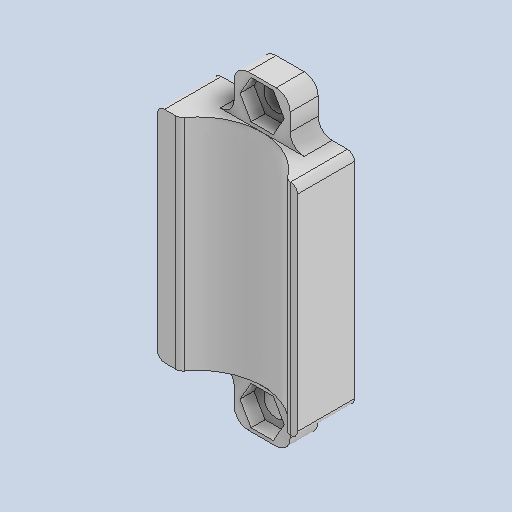
# Autodesk Inventor part: baterry_holder
Saved by Autodesk Inventor 2023 (Build 270158000, 158)
## iProperties
Created: 2023-07-29
Part Number: baterry_holder
Material: Ogólny
Document SubType Name: Modeling
Designer: Kamil
Density: 1 g/cm^3
Appearance: Domyślna
Author: Kamil
Autodesk Inventor part; units mm, degrees
ref_plane "YZ Plane" through (0, 0, 0) normal (1, 0, 0) x (0, 1, 0)
ref_plane "XZ Plane" through (0, 0, 0) normal (0, 1, 0) x (-1, 0, 0)
sketch "Szkic1" plane through (0, 0, 0) normal (0, 0, 1) x (1, 0, 0)
  line L0 (-47.8749, 26.935) -> (-29.4749, 26.935) projected
  line L1 (-47.2702, -7.5558) -> (-30.0796, -7.5558) projected
  line L2 (-29.4749, 23.0223) -> (-29.4749, -7.065)
  line L3 (-47.8749, 23.0223) -> (-47.8749, -7.065)
  line L4 (-47.1734, 27.6365) -> (-30.1764, 27.6365) projected
  line L5 (-47.1749, -7.765) -> (-30.1749, -7.765) projected
  line L6 (-29.4749, 27.6365) -> (-47.8749, 27.6365)
  line L7 (-47.8749, 27.6365) -> (-47.8749, -7.765)
  line L8 (-47.8749, -7.765) -> (-29.4749, -7.765)
  line L9 (-29.4749, -7.765) -> (-29.4749, 27.6365)
  line L10 (-29.4749, 27.6365) -> (-47.8749, 27.6365)
  line L11 (-47.8749, 27.6365) -> (-47.8749, 23.6365)
  line L12 (-47.8749, 23.6365) -> (-29.4749, 23.6365)
  line L13 (-29.4749, 23.6365) -> (-29.4749, 27.6365)
  point P0 (0, 0)
  point P1 (-47.8749, -7.065)
  point P2 (-29.4749, -7.065)
  dimension "d0" = 4
  constraints: 20 end point, 4 parallel, 2 horizontal, 2 perpendicular, 2 vertical, 1 point on line, 4 other
  measures "d0" distance of L11.end L10.end
ref_plane "Płaszczyzna konstrukcyjna1" through (-46.6386, 28.6013, 8.141) normal (0, 0, -1) x (0, 1, 0)
extrude "Wyciągnięcie proste1" add sketch "Szkic1" along normal up to surface (8.141 mm away) contours L12 L9 L2 L8 L5 L7 L3
sketch "Szkic2" plane through (-47.8749, -7.765, 0) normal (0, -1, 0) x (1, 0, 0)
  circle A0 centre (9.2, 13.221) radius 9.2 projected
  line L0 (0, 8.141) -> (18.4, 8.141) projected
  point P0 (47.8749, 0)
  point P1 (16.8703, 8.141)
  point P2 (1.5297, 8.141)
extrude "Wyciągnięcie proste2" cut sketch "Szkic2" against normal through all contours L0 A0 picked at (10.6511, 7.1327)
sketch "Szkic3" plane through (0, 0, 0) normal (0, 0, -1) x (-1, 0, 0)
  line L0 (47.8749, 23.6365) -> (47.8749, -7.765) projected
  line L1 (29.4749, 23.6365) -> (47.8749, 23.6365) projected
  line L2 (29.4749, -7.765) -> (29.4749, 23.6365) projected
  line L3 (47.8749, -7.765) -> (29.4749, -7.765) projected
  line L4 (42.6749, 30.1365) -> (34.6749, 30.1365)
  line L5 (34.6749, 30.1365) -> (34.6749, 23.6365)
  line L6 (34.6749, 23.6365) -> (42.6749, 23.6365)
  line L7 (42.6749, 23.6365) -> (42.6749, 30.1365)
  line L8 (42.6749, -7.765) -> (34.6749, -7.765)
  line L9 (34.6749, -7.765) -> (34.6749, -14.265)
  line L10 (34.6749, -14.265) -> (42.6749, -14.265)
  line L11 (42.6749, -14.265) -> (42.6749, -7.765)
  point P0 (0, 0)
  point P1 (38.6749, 23.6365)
  point P2 (38.6749, 23.6365)
  dimension "d7" = 8
  dimension "d8" = 6.5
  dimension "d9" = 6.5
  constraints: 16 end point, 4 parallel, 2 horizontal, 2 midpoint, 2 perpendicular, 1 coincident, 1 collinear, 1 point on line
  measures "d7" distance of L6.end L5.end
  measures "d8" distance of L5.end L4.end
  measures "d9" distance of L9.end L8.end
extrude "Wyciągnięcie proste3" add sketch "Szkic3" against normal blind 2 contours L1 L5 L4 L7 | L11 L10 L9 L3
sketch "Szkic4" plane through (0, 0, 2) normal (0, 0, 1) x (1, 0, 0)
  line L0 (-34.6749, 23.6365) -> (-34.6749, 30.1365) projected
  line L1 (-34.6749, 30.1365) -> (-42.6749, 30.1365) projected
  line L2 (-42.6749, 30.1365) -> (-42.6749, 23.6365) projected
  line L3 (-34.6749, 23.6365) -> (-42.6749, 23.6365) projected
  line L4 (-42.6749, -7.765) -> (-42.6749, -14.265) projected
  line L5 (-42.6749, -14.265) -> (-34.6749, -14.265) projected
  line L6 (-34.6749, -14.265) -> (-34.6749, -7.765) projected
  line L7 (-42.6749, -7.765) -> (-34.6749, -7.765) projected
  point P0 (0, 0)
  point P1 (-38.6749, 26.8865)
  point P2 (-38.6749, -11.015)
hole "Otwór1" at (-38.6749, 26.8865, 2) at (-38.6749, -11.015, 2) direction (0, 0, -1) diameter 3.5 end through all
sketch "Szkic5" plane through (0, 0, 2) normal (0, 0, 1) x (1, 0, 0)
  circle A0 centre (-38.6749, 26.8865) radius 1.75 projected
  line L0 (-34.6749, 23.6365) -> (-34.6749, 30.1365) projected
  line L1 (-34.6749, 30.1365) -> (-42.6749, 30.1365) projected
  line L2 (-42.6749, 30.1365) -> (-42.6749, 23.6365) projected
  line L3 (-34.6749, 23.6365) -> (-42.6749, 23.6365) projected
  circle A1 centre (-38.6749, -11.015) radius 1.75 projected
  line L4 (-42.6749, -7.765) -> (-42.6749, -14.265) projected
  line L5 (-42.6749, -14.265) -> (-34.6749, -14.265) projected
  line L6 (-34.6749, -14.265) -> (-34.6749, -7.765) projected
  line L7 (-42.6749, -7.765) -> (-34.6749, -7.765) projected
  circle A2 centre (-38.6749, 26.8865) radius 2.75
  circle A3 centre (-38.6749, -11.015) radius 2.75
  line L8 (-37.0872, 29.6365) -> (-35.4995, 26.8865)
  line L9 (-35.4995, 26.8865) -> (-37.0872, 24.1365)
  line L10 (-37.0872, 24.1365) -> (-40.2626, 24.1365)
  line L11 (-40.2626, 24.1365) -> (-41.8503, 26.8865)
  line L12 (-41.8503, 26.8865) -> (-40.2626, 29.6365)
  line L13 (-40.2626, 29.6365) -> (-37.0872, 29.6365)
  line L14 (-40.2626, -13.765) -> (-41.8503, -11.015)
  line L15 (-41.8503, -11.015) -> (-40.2626, -8.265)
  line L16 (-40.2626, -8.265) -> (-37.0872, -8.265)
  line L17 (-37.0872, -8.265) -> (-35.4995, -11.015)
  line L18 (-35.4995, -11.015) -> (-37.0872, -13.765)
  line L19 (-37.0872, -13.765) -> (-40.2626, -13.765)
  point P0 (0, 0)
  point P1 (-38.6749, 29.6365)
  point P2 (-38.6749, -13.765)
  dimension "d19" = 5.5
  dimension "d20" = 5.5
  constraints: 24 end point, 4 coincident, 2 midpoint, 2 vertical alignment, 30 other
extrude "Wyciągnięcie proste4" add sketch "Szkic5" along normal blind 2 contours L3 L2 L1 L0 | L7 L6 L5 L4
sketch "Szkic6" plane through (-47.8749, -7.765, 0) normal (-1, 0, 0) x (0, 0, 1)
  line L0 (8.141, 31.4015) -> (8.141, 0) projected
  line L1 (0, 31.4015) -> (8.141, 31.4015) projected
  line L2 (0, 31.4015) -> (0, 0) projected
  line L3 (0, 0) -> (8.141, 0) projected
  point P0 (0, 7.765)
extrude "Wyciągnięcie proste5" add sketch "Szkic6" along normal blind 1.625
fillet "Zaokrąglenie3" radius 2 8 edges at (-42.6749, 30.1365, 2) (-34.6749, 30.1365, 2) (-34.6749, -14.265, 2) (-42.6749, -14.265, 2) (-42.6749, -7.765, 2) (-34.6749, -7.765, 2) (-34.6749, 23.6365, 2) (-42.6749, 23.6365, 2)
fillet "Zaokrąglenie4" radius 1 4 edges at (-49.4999, -7.765, 4.0705) (-29.4749, -7.765, 4.0705) (-49.4999, 23.6365, 4.0705) (-29.4749, 23.6365, 4.0705)
fillet "Zaokrąglenie5" radius 1 2 edges at (-31.0046, 7.9357, 8.141) (-46.3452, 7.9357, 8.141)
